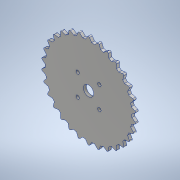
# Autodesk Inventor part: kolo_zebate_duze_fi8
Saved by Autodesk Inventor 2020.3 (Build 243373000, 373)
## iProperties
Created: 2019-08-27
Part Number: kolo_zebate_duze_fi8
Material: Aluminum 6061
Document SubType Name: Modeling
Designer: patry
Density: 2.7 g/cm^3
Appearance: Aluminum - Flat
Mass: 32.4212 g
Surface Area: 106.432 cm^2
Volume: 12.0078 cm^3
Author: patry
Autodesk Inventor part; units mm, degrees
ref_plane "YZ Plane" through (0, 0, 0) normal (1, 0, 0) x (0, 1, 0)
ref_plane "XZ Plane" through (0, 0, 0) normal (0, 1, 0) x (-1, 0, 0)
ref_plane "XY Plane" through (0, 0, 0) normal (0, 0, 1) x (1, 0, 0)
sketch "Szkic2" plane through (0, 0, 0) normal (0, 1, 0) x (-1, 0, 0)
  line L0 (0, 0) -> (-3.9932, -37.9928) construction
  line L1 (0, 0) -> (3.9932, -37.9928) construction
  line L2 (3.9932, -37.9928) -> (-3.9932, -37.9928) construction
  line L3 (0, 0) -> (0, -151) construction
  circle A0 centre (0, 0) radius 38.2021 construction
  line L4 (0, -42.2928) -> (2.7195, -38.1052) construction
  line L5 (0, -42.2928) -> (-2.7195, -38.1052) construction
  circle A1 centre (0, -40.5355) radius 0.9571 construction
  line L6 (2.7195, -38.1052) -> (0.8027, -41.0568)
  line L7 (-2.7195, -38.1052) -> (-0.8027, -41.0568)
  arc A2 (-0.8027, -41.0568) -> (0.8027, -41.0568) centre (0, -40.5355) ccw
  line L8 (-2.7195, -38.1052) -> (5.2625, -37.8379) construction
  arc A3 (2.7195, -38.1052) -> (5.2625, -37.8379) centre (0, 0) ccw
  line L9 (8.7932, -41.3686) -> (5.2625, -37.8379) construction
  line L10 (5.2625, -37.8379) -> (7.751, -40.3265)
  arc A4 (7.751, -40.3265) -> (9.3214, -39.9927) centre (8.4278, -39.6497) ccw
  line L11 (10.5826, -36.7071) -> (9.3214, -39.9927)
  arc A5 (10.5826, -36.7071) -> (13.0144, -35.9169) centre (0, 0) ccw
  line L12 (17.202, -38.6364) -> (13.0144, -35.9169) construction
  line L13 (13.0144, -35.9169) -> (15.966, -37.8337)
  arc A6 (15.966, -37.8337) -> (17.4326, -37.1807) centre (16.4873, -37.031) ccw
  line L14 (17.9832, -33.7047) -> (17.4326, -37.1807)
  arc A7 (17.9832, -33.7047) -> (20.1976, -32.4262) centre (0, 0) ccw
  line L15 (24.8591, -34.2156) -> (20.1976, -32.4262) construction
  line L16 (20.1976, -32.4262) -> (23.4832, -33.6874)
  arc A8 (23.4832, -33.6874) -> (24.782, -32.7438) centre (23.8262, -32.7939) ccw
  line L17 (24.5978, -29.2293) -> (24.782, -32.7438)
  arc A9 (24.5978, -29.2293) -> (26.498, -27.5183) centre (0, 0) ccw
  line L18 (31.4297, -28.2994) -> (26.498, -27.5183) construction
  line L19 (26.498, -27.5183) -> (29.974, -28.0689)
  arc A10 (29.974, -28.0689) -> (31.0482, -26.8758) centre (30.1237, -27.1235) ccw
  line L20 (30.1374, -23.4764) -> (31.0482, -26.8758)
  arc A11 (30.1374, -23.4764) -> (31.6403, -21.4077) centre (0, 0) ccw
  line L21 (36.6267, -21.1464) -> (31.6403, -21.4077) construction
  line L22 (31.6403, -21.4077) -> (35.1548, -21.2235)
  arc A12 (35.1548, -21.2235) -> (35.9576, -19.8332) centre (35.1048, -20.2677) ccw
  line L23 (34.3598, -16.6974) -> (35.9576, -19.8332)
  arc A13 (34.3598, -16.6974) -> (35.3998, -14.3615) centre (0, 0) ccw
  line L24 (40.2229, -13.0692) -> (35.3998, -14.3615) construction
  line L25 (35.3998, -14.3615) -> (38.7993, -13.4507)
  arc A14 (38.7993, -13.4507) -> (39.2954, -11.9238) centre (38.5515, -12.5262) ccw
  line L26 (37.0806, -9.1888) -> (39.2954, -11.9238)
  arc A15 (37.0806, -9.1888) -> (37.6122, -6.6877) centre (0, 0) ccw
  line L27 (42.0611, -4.4208) -> (37.6122, -6.6877) construction
  line L28 (37.6122, -6.6877) -> (40.7479, -5.0899)
  arc A16 (40.7479, -5.0899) -> (40.9158, -3.4933) centre (40.3134, -4.2371) ccw
  line L29 (38.1807, -1.2785) -> (40.9158, -3.4933)
  arc A17 (38.1807, -1.2785) -> (38.1807, 1.2785) centre (0, 0) ccw
  line L30 (42.0611, 4.4208) -> (38.1807, 1.2785) construction
  line L31 (38.1807, 1.2785) -> (40.9158, 3.4933)
  arc A18 (40.9158, 3.4933) -> (40.7479, 5.0899) centre (40.3134, 4.2371) ccw
  line L32 (37.6122, 6.6877) -> (40.7479, 5.0899)
  arc A19 (37.6122, 6.6877) -> (37.0806, 9.1888) centre (0, 0) ccw
  line L33 (40.2229, 13.0692) -> (37.0806, 9.1888) construction
  line L34 (37.0806, 9.1888) -> (39.2954, 11.9238)
  arc A20 (39.2954, 11.9238) -> (38.7993, 13.4507) centre (38.5515, 12.5262) ccw
  line L35 (35.3998, 14.3615) -> (38.7993, 13.4507)
  arc A21 (35.3998, 14.3615) -> (34.3598, 16.6974) centre (0, 0) ccw
  line L36 (36.6267, 21.1464) -> (34.3598, 16.6974) construction
  line L37 (34.3598, 16.6974) -> (35.9576, 19.8332)
  arc A22 (35.9576, 19.8332) -> (35.1548, 21.2235) centre (35.1048, 20.2677) ccw
  line L38 (31.6403, 21.4077) -> (35.1548, 21.2235)
  arc A23 (31.6403, 21.4077) -> (30.1374, 23.4764) centre (0, 0) ccw
  line L39 (31.4297, 28.2994) -> (30.1374, 23.4764) construction
  line L40 (30.1374, 23.4764) -> (31.0482, 26.8758)
  arc A24 (31.0482, 26.8758) -> (29.974, 28.0689) centre (30.1237, 27.1235) ccw
  line L41 (26.498, 27.5183) -> (29.974, 28.0689)
  arc A25 (26.498, 27.5183) -> (24.5978, 29.2293) centre (0, 0) ccw
  line L42 (24.8591, 34.2156) -> (24.5978, 29.2293) construction
  line L43 (24.5978, 29.2293) -> (24.782, 32.7438)
  arc A26 (24.782, 32.7438) -> (23.4832, 33.6874) centre (23.8262, 32.7939) ccw
  line L44 (20.1976, 32.4262) -> (23.4832, 33.6874)
  arc A27 (20.1976, 32.4262) -> (17.9832, 33.7047) centre (0, 0) ccw
  line L45 (17.202, 38.6364) -> (17.9832, 33.7047) construction
  line L46 (17.9832, 33.7047) -> (17.4326, 37.1807)
  arc A28 (17.4326, 37.1807) -> (15.966, 37.8337) centre (16.4873, 37.031) ccw
  line L47 (13.0144, 35.9169) -> (15.966, 37.8337)
  arc A29 (13.0144, 35.9169) -> (10.5826, 36.7071) centre (0, 0) ccw
  line L48 (8.7932, 41.3686) -> (10.5826, 36.7071) construction
  line L49 (10.5826, 36.7071) -> (9.3214, 39.9927)
  arc A30 (9.3214, 39.9927) -> (7.751, 40.3265) centre (8.4278, 39.6497) ccw
  line L50 (5.2625, 37.8379) -> (7.751, 40.3265)
  arc A31 (5.2625, 37.8379) -> (2.7195, 38.1052) centre (0, 0) ccw
  line L51 (0, 42.2928) -> (2.7195, 38.1052) construction
  line L52 (2.7195, 38.1052) -> (0.8027, 41.0568)
  arc A32 (0.8027, 41.0568) -> (-0.8027, 41.0568) centre (0, 40.5355) ccw
  line L53 (-2.7195, 38.1052) -> (-0.8027, 41.0568)
  arc A33 (-2.7195, 38.1052) -> (-5.2625, 37.8379) centre (0, 0) ccw
  line L54 (-8.7932, 41.3686) -> (-5.2625, 37.8379) construction
  line L55 (-5.2625, 37.8379) -> (-7.751, 40.3265)
  arc A34 (-7.751, 40.3265) -> (-9.3214, 39.9927) centre (-8.4278, 39.6497) ccw
  line L56 (-10.5826, 36.7071) -> (-9.3214, 39.9927)
  arc A35 (-10.5826, 36.7071) -> (-13.0144, 35.9169) centre (0, 0) ccw
  line L57 (-17.202, 38.6364) -> (-13.0144, 35.9169) construction
  line L58 (-13.0144, 35.9169) -> (-15.966, 37.8337)
  arc A36 (-15.966, 37.8337) -> (-17.4326, 37.1807) centre (-16.4873, 37.031) ccw
  line L59 (-17.9832, 33.7047) -> (-17.4326, 37.1807)
  arc A37 (-17.9832, 33.7047) -> (-20.1976, 32.4262) centre (0, 0) ccw
  line L60 (-24.8591, 34.2156) -> (-20.1976, 32.4262) construction
  line L61 (-20.1976, 32.4262) -> (-23.4832, 33.6874)
  arc A38 (-23.4832, 33.6874) -> (-24.782, 32.7438) centre (-23.8262, 32.7939) ccw
  line L62 (-24.5978, 29.2293) -> (-24.782, 32.7438)
  arc A39 (-24.5978, 29.2293) -> (-26.498, 27.5183) centre (0, 0) ccw
  line L63 (-31.4297, 28.2994) -> (-26.498, 27.5183) construction
  line L64 (-26.498, 27.5183) -> (-29.974, 28.0689)
  arc A40 (-29.974, 28.0689) -> (-31.0482, 26.8758) centre (-30.1237, 27.1235) ccw
  line L65 (-30.1374, 23.4764) -> (-31.0482, 26.8758)
  arc A41 (-30.1374, 23.4764) -> (-31.6403, 21.4077) centre (0, 0) ccw
  line L66 (-36.6267, 21.1464) -> (-31.6403, 21.4077) construction
  line L67 (-31.6403, 21.4077) -> (-35.1548, 21.2235)
  arc A42 (-35.1548, 21.2235) -> (-35.9576, 19.8332) centre (-35.1048, 20.2677) ccw
  line L68 (-34.3598, 16.6974) -> (-35.9576, 19.8332)
  arc A43 (-34.3598, 16.6974) -> (-35.3998, 14.3615) centre (0, 0) ccw
  line L69 (-40.2229, 13.0692) -> (-35.3998, 14.3615) construction
  line L70 (-35.3998, 14.3615) -> (-38.7993, 13.4507)
  arc A44 (-38.7993, 13.4507) -> (-39.2954, 11.9238) centre (-38.5515, 12.5262) ccw
  line L71 (-37.0806, 9.1888) -> (-39.2954, 11.9238)
  arc A45 (-37.0806, 9.1888) -> (-37.6122, 6.6877) centre (0, 0) ccw
  line L72 (-42.0611, 4.4208) -> (-37.6122, 6.6877) construction
  line L73 (-37.6122, 6.6877) -> (-40.7479, 5.0899)
  arc A46 (-40.7479, 5.0899) -> (-40.9158, 3.4933) centre (-40.3134, 4.2371) ccw
  line L74 (-38.1807, 1.2785) -> (-40.9158, 3.4933)
  arc A47 (-38.1807, 1.2785) -> (-38.1807, -1.2785) centre (0, 0) ccw
  line L75 (-42.0611, -4.4208) -> (-38.1807, -1.2785) construction
  line L76 (-38.1807, -1.2785) -> (-40.9158, -3.4933)
  arc A48 (-40.9158, -3.4933) -> (-40.7479, -5.0899) centre (-40.3134, -4.2371) ccw
  line L77 (-37.6122, -6.6877) -> (-40.7479, -5.0899)
  arc A49 (-37.6122, -6.6877) -> (-37.0806, -9.1888) centre (0, 0) ccw
  line L78 (-40.2229, -13.0692) -> (-37.0806, -9.1888) construction
  line L79 (-37.0806, -9.1888) -> (-39.2954, -11.9238)
  arc A50 (-39.2954, -11.9238) -> (-38.7993, -13.4507) centre (-38.5515, -12.5262) ccw
  line L80 (-35.3998, -14.3615) -> (-38.7993, -13.4507)
  arc A51 (-35.3998, -14.3615) -> (-34.3598, -16.6974) centre (0, 0) ccw
  line L81 (-36.6267, -21.1464) -> (-34.3598, -16.6974) construction
  line L82 (-34.3598, -16.6974) -> (-35.9576, -19.8332)
  arc A52 (-35.9576, -19.8332) -> (-35.1548, -21.2235) centre (-35.1048, -20.2677) ccw
  line L83 (-31.6403, -21.4077) -> (-35.1548, -21.2235)
  arc A53 (-31.6403, -21.4077) -> (-30.1374, -23.4764) centre (0, 0) ccw
  line L84 (-31.4297, -28.2994) -> (-30.1374, -23.4764) construction
  line L85 (-30.1374, -23.4764) -> (-31.0482, -26.8758)
  arc A54 (-31.0482, -26.8758) -> (-29.974, -28.0689) centre (-30.1237, -27.1235) ccw
  line L86 (-26.498, -27.5183) -> (-29.974, -28.0689)
  arc A55 (-26.498, -27.5183) -> (-24.5978, -29.2293) centre (0, 0) ccw
  line L87 (-24.8591, -34.2156) -> (-24.5978, -29.2293) construction
  line L88 (-24.5978, -29.2293) -> (-24.782, -32.7438)
  arc A56 (-24.782, -32.7438) -> (-23.4832, -33.6874) centre (-23.8262, -32.7939) ccw
  line L89 (-20.1976, -32.4262) -> (-23.4832, -33.6874)
  arc A57 (-20.1976, -32.4262) -> (-17.9832, -33.7047) centre (0, 0) ccw
  line L90 (-17.202, -38.6364) -> (-17.9832, -33.7047) construction
  line L91 (-17.9832, -33.7047) -> (-17.4326, -37.1807)
  arc A58 (-17.4326, -37.1807) -> (-15.966, -37.8337) centre (-16.4873, -37.031) ccw
  line L92 (-13.0144, -35.9169) -> (-15.966, -37.8337)
  arc A59 (-13.0144, -35.9169) -> (-10.5826, -36.7071) centre (0, 0) ccw
  line L93 (-8.7932, -41.3686) -> (-10.5826, -36.7071) construction
  line L94 (-10.5826, -36.7071) -> (-9.3214, -39.9927)
  arc A60 (-9.3214, -39.9927) -> (-7.751, -40.3265) centre (-8.4278, -39.6497) ccw
  line L95 (-5.2625, -37.8379) -> (-7.751, -40.3265)
  arc A61 (-5.2625, -37.8379) -> (-2.7195, -38.1052) centre (0, 0) ccw
  dimension "d19" = 7.9864
  dimension "d20" = 3.9932
  dimension "d21" = 12
  dimension "d22" = 4.3
  dimension "d23" = 147
  dimension "d24" = 147
  dimension "d26" = 7.9864
  dimension "d44" = 1.7573
  constraints: 192 end point, 126 point on circle, 62 centre point, 33 point on line, 2 coincident, 2 tangent, 1 concentric, 1 equal length, 1 vertical, 2 other
  measures "d19" distance of L1.end L0.end
  measures "d20" distance from line of L1.end L3
  measures "d21" angle of L1 L0
  measures "d22" distance from line of L2 L4.start
  measures "d23" angle of L3 L4
  measures "d24" angle of L3 L5
  measures "d26" distance of L5.end L8.end
  measures "d44" distance of L4.start point (0, -40.535)
sketch "Szkic3" plane through (0, 0, 0) normal (0, 1, 0) x (-1, 0, 0)
  circle A0 centre (0, 0) radius 13.5 construction
  line L0 (-9.5459, 9.5459) -> (9.5459, 9.5459) construction
  line L1 (9.5459, 9.5459) -> (9.5459, -9.5459) construction
  line L2 (9.5459, -9.5459) -> (-9.5459, -9.5459) construction
  line L3 (-9.5459, -9.5459) -> (-9.5459, 9.5459) construction
  line L4 (-9.5459, 9.5459) -> (9.5459, -9.5459) construction
  line L5 (9.5459, 9.5459) -> (-9.5459, -9.5459) construction
  dimension "d37" = 27
  constraints: 12 end point, 5 coincident, 2 midpoint, 2 parallel, 2 perpendicular, 1 horizontal, 3 other
extrude "Wyciągnięcie proste2" add sketch "Szkic2" along normal blind 2.5
hole "Otwór1" at (-9.5459, 0, -9.5459) at (9.5459, 0, -9.5459) at (9.5459, 0, 9.5459) at (-9.5459, 0, 9.5459) direction (0, 1, 0) diameter 3 end through all
sketch "Szkic4" plane through (0, 0, 0) normal (0, -1, 0) x (1, 0, 0)
  point P0 (0, 0)
  point P1 (0, 0)
  constraints: 1 coincident
hole "Otwór2" at (0, 0, 0) direction (0, 1, 0) diameter 9 end through all
equation "\"d19\" = dl_przeskoku"
equation "\"d20\" = 0.5 * d19"
equation "\"d23\" = kat_zeba"
equation "\"d24\" = kat_zeba"
equation "\"d26\" = dl_przeskoku"
equation "\"kat\" = 360deg"
equation "\"kat_zeba\" = 147deg"
equation "\"wys_zeba\" = 5"
equation "\"odl_osi_zeba\" = 2.366"
equation "\"dl_ogniwa\" = 8.3"
equation "\"dl_przeskoku\" = 7.986415"
